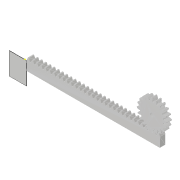
# Autodesk Inventor part: rack and pinion
Saved by Autodesk Inventor 2019 (Build 230136000, 136)
## iProperties
Created: 2020-02-18
Part Number: rack and pinion
Material: Generic
Document SubType Name: Modeling
Designer: hp
Density: 1 g/cm^3
Appearance: Default
Author: hp
Autodesk Inventor part; units mm, degrees
ref_plane "YZ Plane" through (0, 0, 0) normal (1, 0, 0) x (0, 1, 0)
ref_plane "XZ Plane" through (0, 0, 0) normal (0, 1, 0) x (-1, 0, 0)
ref_plane "XY Plane" through (0, 0, 0) normal (0, 0, 1) x (1, 0, 0)
sketch "Sketch1" plane through (-201.5873, -5.3112, -24.2953) normal (-1, 0, 0) x (0, -1, 0)
  point P0 (-5.3112, 24.2953)
sketch "Sketch2" plane through (-199.4341, -5.3112, -4.2953) normal (0, 0, 1) x (1, 0, 0)
  line L0 (0, 0) -> (-65.0744, 0)
  line L1 (-65.0744, 0) -> (-65.0744, -82.528)
  line L2 (-65.0744, -82.528) -> (0, -82.528)
  line L3 (0, -82.528) -> (0, 0)
  point P0 (199.4341, 5.3112)
  constraints: 8 end point, 2 parallel, 1 horizontal, 1 perpendicular
extrude "Extrusion1" add sketch "Sketch2" along normal blind 1
body "Solid1"
